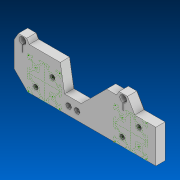
# Autodesk Inventor part: y-rear-V2
Saved by Autodesk Inventor 2021 (Build 250183000, 183)
## iProperties
Created: 2021-03-09
Part Number: y-rear-V2
Material: Generic
Document SubType Name: Modeling
Designer: Alex
Density: 1 g/cm^3
Appearance: Default
Author: Alex
## iProperties of the stored document _3DPrint.ipt
Created: 2021-03-16
Part Number: _3DPrint
Material: Generic
Document SubType Name: Modeling
Designer: Alex
Density: 1 g/cm^3
Appearance: Default
Author: Alex
Autodesk Inventor part; units mm, degrees
ref_plane "YZ Plane" through (0, 0, 0) normal (1, 0, 0) x (0, 1, 0)
ref_plane "XZ Plane" through (0, 0, 0) normal (0, 1, 0) x (-1, 0, 0)
ref_plane "XY Plane" through (0, 0, 0) normal (0, 0, 1) x (1, 0, 0)
sketch "v_slot_locations" plane through (0, 0, 0) normal (0, 0, 1) x (1, 0, 0)
  circle A0 centre (10, 10) radius 2.3 construction
  line L0 (13.9, 12.8393) -> (13.9, 7.1607) construction
  line L1 (12.8393, 13.9) -> (13.9, 12.8393) construction
  line L2 (7.1607, 13.9) -> (12.8393, 13.9) construction
  line L3 (3.7607, 17.3) -> (7.1607, 13.9) construction
  line L4 (1.8, 17.3) -> (3.7607, 17.3) construction
  line L5 (1.8, 22.7) -> (1.8, 17.3) construction
  line L6 (17.3, 1.8) -> (22.7, 1.8) construction
  line L7 (17.3, 3.7607) -> (17.3, 1.8) construction
  line L8 (13.9, 7.1607) -> (17.3, 3.7607) construction
  line L9 (0, 14.58) -> (0, 25.42) construction
  line L10 (1.185, 13.395) -> (0, 14.58) construction
  line L11 (1.8, 13.395) -> (1.185, 13.395) construction
  line L12 (1.8, 15.5) -> (1.8, 13.395) construction
  line L13 (3.4393, 15.5) -> (1.8, 15.5) construction
  line L14 (6.1, 12.8393) -> (3.4393, 15.5) construction
  line L15 (6.1, 10.21) -> (6.1, 12.8393) construction
  line L16 (6.31, 10) -> (6.1, 10.21) construction
  line L17 (6.1, 9.79) -> (6.31, 10) construction
  line L18 (6.1, 7.1607) -> (6.1, 9.79) construction
  line L19 (3.4393, 4.5) -> (6.1, 7.1607) construction
  line L20 (1.8, 4.5) -> (3.4393, 4.5) construction
  line L21 (1.8, 6.605) -> (1.8, 4.5) construction
  line L22 (1.185, 6.605) -> (1.8, 6.605) construction
  line L23 (0, 5.42) -> (1.185, 6.605) construction
  line L24 (0, 1.5) -> (0, 5.42) construction
  arc A1 (0, 1.5) -> (1.5, 0) centre (1.5, 1.5) ccw construction
  line L25 (5.42, 0) -> (1.5, 0) construction
  line L26 (6.605, 1.185) -> (5.42, 0) construction
  line L27 (6.605, 1.8) -> (6.605, 1.185) construction
  line L28 (4.5, 1.8) -> (6.605, 1.8) construction
  line L29 (4.5, 3.4393) -> (4.5, 1.8) construction
  line L30 (7.1607, 6.1) -> (4.5, 3.4393) construction
  line L31 (9.79, 6.1) -> (7.1607, 6.1) construction
  line L32 (10, 6.31) -> (9.79, 6.1) construction
  line L33 (10.21, 6.1) -> (10, 6.31) construction
  line L34 (12.8393, 6.1) -> (10.21, 6.1) construction
  line L35 (15.5, 3.4393) -> (12.8393, 6.1) construction
  line L36 (15.5, 1.8) -> (15.5, 3.4393) construction
  line L37 (13.395, 1.8) -> (15.5, 1.8) construction
  line L38 (13.395, 1.185) -> (13.395, 1.8) construction
  line L39 (14.58, 0) -> (13.395, 1.185) construction
  line L40 (25.42, 0) -> (14.58, 0) construction
  line L41 (0, 1.5) -> (0, 0) construction
  line L42 (0, 0) -> (1.5, 0) construction
  line L43 (0, 20) -> (40, 20) construction
  line L44 (20, 0) -> (20, 40) construction
  line L45 (33.9, 10.21) -> (33.9, 12.8393) construction
  line L46 (32.8393, 13.9) -> (27.1607, 13.9) construction
  line L47 (33.69, 10) -> (33.9, 10.21) construction
  line L48 (33.9, 9.79) -> (33.69, 10) construction
  line L49 (27.1607, 13.9) -> (26.1, 12.8393) construction
  line L50 (33.9, 7.1607) -> (33.9, 9.79) construction
  circle A2 centre (30, 10) radius 2.3 construction
  line L51 (30.21, 6.1) -> (32.8393, 6.1) construction
  line L52 (26.1, 12.8393) -> (26.1, 7.1607) construction
  line L53 (30, 6.31) -> (30.21, 6.1) construction
  line L54 (29.79, 6.1) -> (30, 6.31) construction
  line L55 (27.1607, 6.1) -> (29.79, 6.1) construction
  line L56 (33.9, 12.8393) -> (36.5607, 15.5) construction
  line L57 (38.2, 13.395) -> (38.815, 13.395) construction
  line L58 (36.2393, 17.3) -> (32.8393, 13.9) construction
  line L59 (38.2, 15.5) -> (38.2, 13.395) construction
  line L60 (38.815, 13.395) -> (40, 14.58) construction
  line L61 (38.2, 17.3) -> (36.2393, 17.3) construction
  line L62 (38.2, 22.7) -> (38.2, 17.3) construction
  line L63 (40, 14.58) -> (40, 25.42) construction
  line L64 (36.5607, 15.5) -> (38.2, 15.5) construction
  line L65 (38.815, 6.605) -> (38.2, 6.605) construction
  line L66 (40, 5.42) -> (38.815, 6.605) construction
  line L67 (36.5607, 4.5) -> (33.9, 7.1607) construction
  line L68 (38.2, 6.605) -> (38.2, 4.5) construction
  line L69 (38.2, 4.5) -> (36.5607, 4.5) construction
  line L70 (32.8393, 6.1) -> (35.5, 3.4393) construction
  line L71 (40, 1.5) -> (40, 5.42) construction
  line L72 (35.5, 3.4393) -> (35.5, 1.8) construction
  line L73 (35.5, 1.8) -> (33.395, 1.8) construction
  line L74 (33.395, 1.8) -> (33.395, 1.185) construction
  line L75 (33.395, 1.185) -> (34.58, 0) construction
  line L76 (34.58, 0) -> (38.5, 0) construction
  arc A3 (38.5, 0) -> (40, 1.5) centre (38.5, 1.5) ccw construction
  line L77 (22.7, 3.7607) -> (22.7, 1.8) construction
  line L78 (26.1, 7.1607) -> (22.7, 3.7607) construction
  line L79 (25.42, 0) -> (26.605, 1.185) construction
  line L80 (24.5, 3.4393) -> (27.1607, 6.1) construction
  line L81 (24.5, 1.8) -> (24.5, 3.4393) construction
  line L82 (26.605, 1.8) -> (24.5, 1.8) construction
  line L83 (26.605, 1.185) -> (26.605, 1.8) construction
  line L84 (6.1, 29.79) -> (6.1, 27.1607) construction
  line L85 (7.1607, 26.1) -> (12.8393, 26.1) construction
  line L86 (6.31, 30) -> (6.1, 29.79) construction
  line L87 (6.1, 30.21) -> (6.31, 30) construction
  line L88 (12.8393, 26.1) -> (13.9, 27.1607) construction
  line L89 (6.1, 32.8393) -> (6.1, 30.21) construction
  circle A4 centre (10, 30) radius 2.3 construction
  line L90 (9.79, 33.9) -> (7.1607, 33.9) construction
  line L91 (13.9, 27.1607) -> (13.9, 32.8393) construction
  line L92 (10, 33.69) -> (9.79, 33.9) construction
  line L93 (10.21, 33.9) -> (10, 33.69) construction
  line L94 (12.8393, 33.9) -> (10.21, 33.9) construction
  line L95 (6.1, 27.1607) -> (3.4393, 24.5) construction
  line L96 (1.8, 26.605) -> (1.185, 26.605) construction
  line L97 (3.7607, 22.7) -> (7.1607, 26.1) construction
  line L98 (1.8, 24.5) -> (1.8, 26.605) construction
  line L99 (1.185, 26.605) -> (0, 25.42) construction
  line L100 (1.8, 22.7) -> (3.7607, 22.7) construction
  line L101 (3.4393, 24.5) -> (1.8, 24.5) construction
  line L102 (1.185, 33.395) -> (1.8, 33.395) construction
  line L103 (0, 34.58) -> (1.185, 33.395) construction
  line L104 (3.4393, 35.5) -> (6.1, 32.8393) construction
  line L105 (1.8, 33.395) -> (1.8, 35.5) construction
  line L106 (1.8, 35.5) -> (3.4393, 35.5) construction
  line L107 (7.1607, 33.9) -> (4.5, 36.5607) construction
  line L108 (0, 38.5) -> (0, 34.58) construction
  line L109 (4.5, 36.5607) -> (4.5, 38.2) construction
  line L110 (4.5, 38.2) -> (6.605, 38.2) construction
  line L111 (6.605, 38.2) -> (6.605, 38.815) construction
  line L112 (6.605, 38.815) -> (5.42, 40) construction
  line L113 (5.42, 40) -> (1.5, 40) construction
  arc A5 (1.5, 40) -> (0, 38.5) centre (1.5, 38.5) ccw construction
  line L114 (17.3, 38.2) -> (22.7, 38.2) construction
  line L115 (17.3, 36.2393) -> (17.3, 38.2) construction
  line L116 (13.9, 32.8393) -> (17.3, 36.2393) construction
  line L117 (14.58, 40) -> (13.395, 38.815) construction
  line L118 (15.5, 36.5607) -> (12.8393, 33.9) construction
  line L119 (15.5, 38.2) -> (15.5, 36.5607) construction
  line L120 (13.395, 38.2) -> (15.5, 38.2) construction
  line L121 (25.42, 40) -> (14.58, 40) construction
  line L122 (13.395, 38.815) -> (13.395, 38.2) construction
  line L123 (38.815, 26.605) -> (40, 25.42) construction
  line L124 (38.2, 26.605) -> (38.815, 26.605) construction
  line L125 (38.2, 24.5) -> (38.2, 26.605) construction
  line L126 (36.5607, 24.5) -> (38.2, 24.5) construction
  line L127 (38.2, 22.7) -> (36.2393, 22.7) construction
  line L128 (36.2393, 22.7) -> (32.8393, 26.1) construction
  line L129 (33.9, 27.1607) -> (36.5607, 24.5) construction
  line L130 (33.9, 29.79) -> (33.9, 27.1607) construction
  line L131 (32.8393, 26.1) -> (27.1607, 26.1) construction
  circle A6 centre (30, 30) radius 2.3 construction
  line L132 (33.9, 30.21) -> (33.69, 30) construction
  line L133 (33.69, 30) -> (33.9, 29.79) construction
  line L134 (33.9, 32.8393) -> (33.9, 30.21) construction
  line L135 (38.815, 33.395) -> (38.2, 33.395) construction
  line L136 (40, 34.58) -> (38.815, 33.395) construction
  line L137 (40, 38.5) -> (40, 34.58) construction
  line L138 (38.2, 33.395) -> (38.2, 35.5) construction
  line L139 (38.2, 35.5) -> (36.5607, 35.5) construction
  arc A7 (40, 38.5) -> (38.5, 40) centre (38.5, 38.5) ccw construction
  line L140 (34.58, 40) -> (38.5, 40) construction
  line L141 (33.395, 38.815) -> (34.58, 40) construction
  line L142 (33.395, 38.2) -> (33.395, 38.815) construction
  line L143 (35.5, 38.2) -> (33.395, 38.2) construction
  line L144 (35.5, 36.5607) -> (35.5, 38.2) construction
  line L145 (32.8393, 33.9) -> (35.5, 36.5607) construction
  line L146 (36.5607, 35.5) -> (33.9, 32.8393) construction
  line L147 (30.21, 33.9) -> (32.8393, 33.9) construction
  line L148 (29.79, 33.9) -> (30, 33.69) construction
  line L149 (30, 33.69) -> (30.21, 33.9) construction
  line L150 (27.1607, 33.9) -> (29.79, 33.9) construction
  line L151 (24.5, 36.5607) -> (27.1607, 33.9) construction
  line L152 (26.605, 38.815) -> (26.605, 38.2) construction
  line L153 (25.42, 40) -> (26.605, 38.815) construction
  line L154 (26.605, 38.2) -> (24.5, 38.2) construction
  line L155 (24.5, 38.2) -> (24.5, 36.5607) construction
  line L156 (22.7, 36.2393) -> (22.7, 38.2) construction
  line L157 (26.1, 32.8393) -> (22.7, 36.2393) construction
  line L158 (26.1, 27.1607) -> (26.1, 32.8393) construction
  line L159 (27.1607, 26.1) -> (26.1, 27.1607) construction
  line L160 (-96.9, 10.21) -> (-96.9, 12.8393) construction
  line L161 (-95.8393, 13.9) -> (-90.1607, 13.9) construction
  line L162 (-96.69, 10) -> (-96.9, 10.21) construction
  line L163 (-96.9, 9.79) -> (-96.69, 10) construction
  line L164 (-90.1607, 13.9) -> (-89.1, 12.8393) construction
  line L165 (-96.9, 7.1607) -> (-96.9, 9.79) construction
  circle A8 centre (-93, 10) radius 2.3 construction
  line L166 (-93.21, 6.1) -> (-95.8393, 6.1) construction
  line L167 (-89.1, 12.8393) -> (-89.1, 7.1607) construction
  line L168 (-93, 6.31) -> (-93.21, 6.1) construction
  line L169 (-92.79, 6.1) -> (-93, 6.31) construction
  line L170 (-90.1607, 6.1) -> (-92.79, 6.1) construction
  line L171 (-96.9, 12.8393) -> (-99.5607, 15.5) construction
  line L172 (-101.2, 13.395) -> (-101.815, 13.395) construction
  line L173 (-99.2393, 17.3) -> (-95.8393, 13.9) construction
  line L174 (-101.2, 15.5) -> (-101.2, 13.395) construction
  line L175 (-101.815, 13.395) -> (-103, 14.58) construction
  line L176 (-101.2, 17.3) -> (-99.2393, 17.3) construction
  line L177 (-101.2, 22.7) -> (-101.2, 17.3) construction
  line L178 (-103, 14.58) -> (-103, 25.42) construction
  line L179 (-99.5607, 15.5) -> (-101.2, 15.5) construction
  line L180 (-101.815, 6.605) -> (-101.2, 6.605) construction
  line L181 (-103, 5.42) -> (-101.815, 6.605) construction
  line L182 (-99.5607, 4.5) -> (-96.9, 7.1607) construction
  line L183 (-101.2, 6.605) -> (-101.2, 4.5) construction
  line L184 (-101.2, 4.5) -> (-99.5607, 4.5) construction
  line L185 (-95.8393, 6.1) -> (-98.5, 3.4393) construction
  line L186 (-103, 1.5) -> (-103, 5.42) construction
  line L187 (-98.5, 3.4393) -> (-98.5, 1.8) construction
  line L188 (-98.5, 1.8) -> (-96.395, 1.8) construction
  line L189 (-96.395, 1.8) -> (-96.395, 1.185) construction
  line L190 (-96.395, 1.185) -> (-97.58, 0) construction
  line L191 (-97.58, 0) -> (-101.5, 0) construction
  arc A9 (-103, 1.5) -> (-101.5, 0) centre (-101.5, 1.5) ccw construction
  line L192 (-85.7, 1.8) -> (-80.3, 1.8) construction
  line L193 (-85.7, 3.7607) -> (-85.7, 1.8) construction
  line L194 (-89.1, 7.1607) -> (-85.7, 3.7607) construction
  line L195 (-88.42, 0) -> (-89.605, 1.185) construction
  line L196 (-87.5, 3.4393) -> (-90.1607, 6.1) construction
  line L197 (-87.5, 1.8) -> (-87.5, 3.4393) construction
  line L198 (-89.605, 1.8) -> (-87.5, 1.8) construction
  line L199 (-77.58, 0) -> (-88.42, 0) construction
  line L200 (-89.605, 1.185) -> (-89.605, 1.8) construction
  line L201 (-103, 1.5) -> (-103, 0) construction
  line L202 (-103, 0) -> (-101.5, 0) construction
  line L203 (-103, 20) -> (-63, 20) construction
  line L204 (-83, 0) -> (-83, 40) construction
  line L205 (-64.185, 13.395) -> (-63, 14.58) construction
  line L206 (-64.8, 13.395) -> (-64.185, 13.395) construction
  line L207 (-64.8, 15.5) -> (-64.8, 13.395) construction
  line L208 (-66.4393, 15.5) -> (-64.8, 15.5) construction
  line L209 (-64.8, 17.3) -> (-66.7607, 17.3) construction
  line L210 (-66.7607, 17.3) -> (-70.1607, 13.9) construction
  line L211 (-69.1, 12.8393) -> (-66.4393, 15.5) construction
  line L212 (-69.1, 10.21) -> (-69.1, 12.8393) construction
  line L213 (-70.1607, 13.9) -> (-75.8393, 13.9) construction
  circle A10 centre (-73, 10) radius 2.3 construction
  line L214 (-69.1, 9.79) -> (-69.31, 10) construction
  line L215 (-69.31, 10) -> (-69.1, 10.21) construction
  line L216 (-69.1, 7.1607) -> (-69.1, 9.79) construction
  line L217 (-64.185, 6.605) -> (-64.8, 6.605) construction
  line L218 (-63, 5.42) -> (-64.185, 6.605) construction
  line L219 (-63, 1.5) -> (-63, 5.42) construction
  line L220 (-64.8, 6.605) -> (-64.8, 4.5) construction
  line L221 (-64.8, 4.5) -> (-66.4393, 4.5) construction
  arc A11 (-64.5, 0) -> (-63, 1.5) centre (-64.5, 1.5) ccw construction
  line L222 (-68.42, 0) -> (-64.5, 0) construction
  line L223 (-69.605, 1.185) -> (-68.42, 0) construction
  line L224 (-69.605, 1.8) -> (-69.605, 1.185) construction
  line L225 (-67.5, 1.8) -> (-69.605, 1.8) construction
  line L226 (-67.5, 3.4393) -> (-67.5, 1.8) construction
  line L227 (-70.1607, 6.1) -> (-67.5, 3.4393) construction
  line L228 (-66.4393, 4.5) -> (-69.1, 7.1607) construction
  line L229 (-72.79, 6.1) -> (-70.1607, 6.1) construction
  line L230 (-73.21, 6.1) -> (-73, 6.31) construction
  line L231 (-73, 6.31) -> (-72.79, 6.1) construction
  line L232 (-75.8393, 6.1) -> (-73.21, 6.1) construction
  line L233 (-78.5, 3.4393) -> (-75.8393, 6.1) construction
  line L234 (-76.395, 1.185) -> (-76.395, 1.8) construction
  line L235 (-77.58, 0) -> (-76.395, 1.185) construction
  line L236 (-76.395, 1.8) -> (-78.5, 1.8) construction
  line L237 (-78.5, 1.8) -> (-78.5, 3.4393) construction
  line L238 (-80.3, 3.7607) -> (-80.3, 1.8) construction
  line L239 (-76.9, 7.1607) -> (-80.3, 3.7607) construction
  line L240 (-76.9, 12.8393) -> (-76.9, 7.1607) construction
  line L241 (-75.8393, 13.9) -> (-76.9, 12.8393) construction
  line L242 (-63, 14.58) -> (-63, 25.42) construction
  line L243 (-64.8, 22.7) -> (-64.8, 17.3) construction
  line L244 (-80.3, 36.2393) -> (-80.3, 38.2) construction
  line L245 (-78.5, 38.2) -> (-78.5, 36.5607) construction
  line L246 (-77.58, 40) -> (-76.395, 38.815) construction
  line L247 (-76.395, 38.815) -> (-76.395, 38.2) construction
  line L248 (-76.395, 38.2) -> (-78.5, 38.2) construction
  line L249 (-76.9, 32.8393) -> (-80.3, 36.2393) construction
  line L250 (-78.5, 36.5607) -> (-75.8393, 33.9) construction
  line L251 (-70.1607, 26.1) -> (-75.8393, 26.1) construction
  circle A12 centre (-73, 30) radius 2.3 construction
  line L252 (-72.79, 33.9) -> (-70.1607, 33.9) construction
  line L253 (-73, 33.69) -> (-72.79, 33.9) construction
  line L254 (-73.21, 33.9) -> (-73, 33.69) construction
  line L255 (-75.8393, 33.9) -> (-73.21, 33.9) construction
  line L256 (-76.9, 27.1607) -> (-76.9, 32.8393) construction
  line L257 (-75.8393, 26.1) -> (-76.9, 27.1607) construction
  line L258 (-63, 38.5) -> (-63, 34.58) construction
  line L259 (-67.5, 36.5607) -> (-67.5, 38.2) construction
  line L260 (-67.5, 38.2) -> (-69.605, 38.2) construction
  line L261 (-69.605, 38.2) -> (-69.605, 38.815) construction
  arc A13 (-63, 38.5) -> (-64.5, 40) centre (-64.5, 38.5) ccw construction
  line L262 (-68.42, 40) -> (-64.5, 40) construction
  line L263 (-69.605, 38.815) -> (-68.42, 40) construction
  line L264 (-69.1, 32.8393) -> (-69.1, 30.21) construction
  line L265 (-64.185, 33.395) -> (-64.8, 33.395) construction
  line L266 (-63, 34.58) -> (-64.185, 33.395) construction
  line L267 (-66.4393, 35.5) -> (-69.1, 32.8393) construction
  line L268 (-64.8, 35.5) -> (-66.4393, 35.5) construction
  line L269 (-64.8, 33.395) -> (-64.8, 35.5) construction
  line L270 (-70.1607, 33.9) -> (-67.5, 36.5607) construction
  line L271 (-64.8, 22.7) -> (-66.7607, 22.7) construction
  line L272 (-66.7607, 22.7) -> (-70.1607, 26.1) construction
  line L273 (-69.31, 30) -> (-69.1, 29.79) construction
  line L274 (-69.1, 30.21) -> (-69.31, 30) construction
  line L275 (-69.1, 29.79) -> (-69.1, 27.1607) construction
  line L276 (-69.1, 27.1607) -> (-66.4393, 24.5) construction
  line L277 (-66.4393, 24.5) -> (-64.8, 24.5) construction
  line L278 (-64.8, 24.5) -> (-64.8, 26.605) construction
  line L279 (-64.185, 26.605) -> (-63, 25.42) construction
  line L280 (-64.8, 26.605) -> (-64.185, 26.605) construction
  line L281 (-95.8393, 26.1) -> (-90.1607, 26.1) construction
  line L282 (-90.1607, 26.1) -> (-89.1, 27.1607) construction
  line L283 (-96.9, 29.79) -> (-96.9, 27.1607) construction
  line L284 (-96.69, 30) -> (-96.9, 29.79) construction
  circle A14 centre (-93, 30) radius 2.3 construction
  line L285 (-89.1, 27.1607) -> (-89.1, 32.8393) construction
  line L286 (-92.79, 33.9) -> (-93, 33.69) construction
  line L287 (-90.1607, 33.9) -> (-92.79, 33.9) construction
  line L288 (-96.9, 30.21) -> (-96.69, 30) construction
  line L289 (-93, 33.69) -> (-93.21, 33.9) construction
  line L290 (-96.9, 32.8393) -> (-96.9, 30.21) construction
  line L291 (-96.9, 27.1607) -> (-99.5607, 24.5) construction
  line L292 (-99.2393, 22.7) -> (-95.8393, 26.1) construction
  line L293 (-87.5, 36.5607) -> (-90.1607, 33.9) construction
  line L294 (-89.1, 32.8393) -> (-85.7, 36.2393) construction
  line L295 (-98.5, 38.2) -> (-96.395, 38.2) construction
  line L296 (-96.395, 38.2) -> (-96.395, 38.815) construction
  line L297 (-96.395, 38.815) -> (-97.58, 40) construction
  line L298 (-101.2, 35.5) -> (-99.5607, 35.5) construction
  line L299 (-98.5, 36.5607) -> (-98.5, 38.2) construction
  line L300 (-97.58, 40) -> (-101.5, 40) construction
  line L301 (-101.2, 33.395) -> (-101.2, 35.5) construction
  line L302 (-103, 34.58) -> (-101.815, 33.395) construction
  line L303 (-101.815, 33.395) -> (-101.2, 33.395) construction
  line L304 (-95.8393, 33.9) -> (-98.5, 36.5607) construction
  line L305 (-99.5607, 35.5) -> (-96.9, 32.8393) construction
  line L306 (-93.21, 33.9) -> (-95.8393, 33.9) construction
  line L307 (-103, 38.5) -> (-103, 34.58) construction
  arc A15 (-101.5, 40) -> (-103, 38.5) centre (-101.5, 38.5) ccw construction
  line L308 (-89.605, 38.815) -> (-89.605, 38.2) construction
  line L309 (-88.42, 40) -> (-89.605, 38.815) construction
  line L310 (-89.605, 38.2) -> (-87.5, 38.2) construction
  line L311 (-87.5, 38.2) -> (-87.5, 36.5607) construction
  line L312 (-77.58, 40) -> (-88.42, 40) construction
  line L313 (-85.7, 36.2393) -> (-85.7, 38.2) construction
  line L314 (-85.7, 38.2) -> (-80.3, 38.2) construction
  line L315 (-101.2, 26.605) -> (-101.815, 26.605) construction
  line L316 (-101.815, 26.605) -> (-103, 25.42) construction
  line L317 (-101.2, 24.5) -> (-101.2, 26.605) construction
  line L318 (-99.5607, 24.5) -> (-101.2, 24.5) construction
  line L319 (-101.2, 22.7) -> (-99.2393, 22.7) construction
  point P0 (0, 0)
  dimension "d3" = 1.5
  dimension "d4" = 4.6
  dimension "d5" = 1.5
  dimension "d7" = 45
  dimension "d8" = 2.105
  dimension "d9" = 1.6393
  dimension "d10" = 1.185
  dimension "d11" = 45
  dimension "d12" = 0.615
  dimension "d13" = 45
  dimension "d16" = 135
  dimension "d17" = 135
  dimension "d18" = 45
  dimension "d19" = 1.5
  dimension "d20" = 2.6293
  dimension "d21" = 2.6293
  dimension "d23" = 45
  dimension "d24" = 2.105
  dimension "d25" = 10.84
  dimension "d26" = 135
  dimension "d27" = 135
  dimension "d28" = 2.6607
  dimension "d29" = 45
  dimension "d30" = 1.185
  dimension "d33" = 0.21
  dimension "d34" = 1.5
  dimension "d35" = 3.9
  dimension "d36" = 3.9
  dimension "d37" = 135
  dimension "d38" = 1.0607
  dimension "d39" = 1.185
  dimension "d40" = 0.615
  dimension "d41" = 1.6393
  dimension "d42" = 1.8
  dimension "d43" = 0.21
  dimension "d44" = 135
  dimension "d45" = 5.4
  dimension "d46" = 1.9607
  dimension "d47" = 1.8
  dimension "d49" = 5.4
  dimension "d50" = 1.8
  dimension "d51" = 40
  dimension "d52" = 40
  dimension "d98" = 13.395
  dimension "d99" = 10
  dimension "d100" = 10
  dimension "d101" = 6.605
  dimension "d102" = 10
  dimension "d103" = 13.395
  dimension "d104" = 1.5
  dimension "d105" = 4.6
  dimension "d106" = 1.5
  dimension "d107" = 45
  dimension "d108" = 2.105
  dimension "d109" = 1.6393
  dimension "d110" = 1.185
  dimension "d111" = 45
  dimension "d112" = 0.615
  dimension "d113" = 45
  dimension "d114" = 135
  dimension "d115" = 135
  dimension "d116" = 45
  dimension "d117" = 1.5
  dimension "d118" = 2.6293
  constraints: 640 end point, 244 symmetric about line, 30 vertical, 28 horizontal, 18 equal length, 16 centre point, 16 point on circle, 7 collinear, 4 midpoint, 4 tangent, 2 perpendicular, 1 coincident, 12 other
  measures "d3" radius of A1
  measures "d4" diameter of A0
  measures "d5" distance between parallel lines of L30 L19
  measures "d7" angle of L25 L26
  measures "d8" distance of L29.end L28.end
  measures "d9" distance of L30.end L29.end
  measures "d10" horizontal distance of L27.end L26.end
  measures "d11" angle of L24 L23
  measures "d12" distance of L28.end L27.end
  measures "d13" angle of L30 L29
  measures "d16" angle of L18 L17
  measures "d17" angle of L15 L16
  measures "d18" angle of L0 L1
  measures "d19" distance between parallel lines of L3 L14
  measures "d20" distance of L18.start L17.start
  measures "d21" distance of L15.start L15.end
  measures "d23" angle of L11 L10
  measures "d24" distance of L12.start L11.start
  measures "d25" distance of L10.end L9.end
  measures "d26" angle of L31 L32
  measures "d27" angle of L34 L33
  measures "d28" horizontal distance of L31.end L30.end
  measures "d29" angle of L40 L39
  measures "d30" horizontal distance of L39.start L39.end
  measures "d33" horizontal distance of L32.start L31.start
  measures "d34" distance between parallel lines of L8 L35
  measures "d35" distance from line of L0 A0.centre
  measures "d36" distance from line of L2 A0.centre
  measures "d37" angle of L35 L36
  measures "d38" horizontal distance of L2.end L1.end
  measures "d39" horizontal distance of L11.end L10.end
  measures "d40" distance of L11.start L11.end
  measures "d41" distance of L14.end L12.start
  measures "d42" distance between parallel lines of L13 L4
  measures "d43" horizontal distance of L16.start L15.start
  measures "d44" angle of L2 L3
  measures "d45" distance of L6.start L6.end
  measures "d46" distance of L7.start L6.start
  measures "d47" distance between parallel lines of L7 L36
  measures "d49" distance of L5.start L4.start
  measures "d50" distance between parallel lines of L9 L5
  measures "d51" distance of L43.start L43.end
  measures "d52" distance of L44.start L44.end
  measures "d98" distance between parallel lines of L38 L24
  measures "d99" distance from line of A0.centre L24
  measures "d100" distance from line of L32.start L24
  measures "d101" distance between parallel lines of L27 L24
  measures "d102" distance from line of A0.centre L25
  measures "d103" distance between parallel lines of L11 L25
  measures "d104" radius of A9
  measures "d105" diameter of A8
  measures "d106" distance between parallel lines of L185 L182
  measures "d107" angle of L191 L190
  measures "d108" distance of L187.end L188.end
  measures "d109" distance of L185.end L187.end
  measures "d110" horizontal distance of L189.end L190.end
  measures "d111" angle of L186 L181
  measures "d112" distance of L188.end L189.end
  measures "d113" angle of L185 L187
  measures "d114" angle of L165 L163
  measures "d115" angle of L160 L162
  measures "d116" angle of L167 L164
  measures "d117" distance between parallel lines of L173 L171
  measures "d118" distance of L165.start L165.end
sketch "Sketch2" plane through (0, 0, 0) normal (0, 0, 1) x (1, 0, 0)
  line L0 (-103, 0) -> (50, 0)
  line L1 (50, 0) -> (50, 40)
  line L2 (50, 40) -> (24.8564, 40)
  line L3 (24.8564, 40) -> (16.1962, 55)
  line L4 (16.1962, 55) -> (6.1962, 55)
  line L5 (6.1962, 55) -> (3.3094, 50)
  line L6 (3.3094, 50) -> (-100.9171, 50)
  line L7 (-100.9171, 50) -> (-103.8038, 55)
  line L8 (-103.8038, 55) -> (-113.8038, 55)
  line L9 (-113.8038, 55) -> (-119, 46)
  line L10 (-119, 46) -> (-119, 16)
  line L11 (-119, 16) -> (-103, 0)
  line L12 (-152.8, 0) -> (83.8, 0) projected
  circle A0 centre (-73, 30) radius 2.3 construction
  circle A1 centre (-93, 10) radius 2.3 construction
  circle A2 centre (10, 10) radius 2.3 construction
  circle A3 centre (30, 30) radius 2.3 construction
  arc A4 (-108.4288, 45.9423) -> (-109.1788, 45.9423) centre (-108.8038, 50) ccw
  arc A5 (11.5712, 45.9423) -> (10.8212, 45.9423) centre (11.1962, 50) ccw
  line L13 (-108.8038, 55) -> (-108.8038, 50) construction
  line L14 (11.1962, 55) -> (11.1962, 50) construction
  line L15 (-109.1788, 45.9423) -> (-109.1788, 37.9423)
  line L16 (-109.1788, 37.9423) -> (-108.4288, 37.9423)
  line L17 (-108.4288, 37.9423) -> (-108.4288, 45.9423)
  line L18 (10.8212, 45.9423) -> (10.8212, 37.9423)
  line L19 (10.8212, 37.9423) -> (11.5712, 37.9423)
  line L20 (11.5712, 37.9423) -> (11.5712, 45.9423)
  line L21 (40, 14.58) -> (40, 25.42) construction
  line L22 (25.42, 40) -> (14.58, 40) construction
  line L23 (-103, 1.5) -> (-103, 0) construction
  line L24 (-48.8038, 50) -> (-48.8038, 0) construction
  line L25 (-63.9171, 50) -> (-58.8038, 20)
  line L26 (-58.8038, 20) -> (-38.8038, 20)
  line L27 (-38.8038, 20) -> (-8.8038, 50)
  circle A6 centre (-53.8038, 10) radius 1.7
  circle A7 centre (-43.8038, 10) radius 1.7
  line L28 (-53.8038, 10) -> (-43.8038, 10) construction
  circle A8 centre (-93, 10) radius 2.75
  circle A9 centre (-73, 30) radius 2.75
  circle A10 centre (10, 10) radius 2.75
  circle A11 centre (30, 30) radius 2.75
  point P0 (0, 0)
  dimension "d154" = 5
  dimension "d155" = 8.15
  dimension "d156" = 0.75
  dimension "d157" = 8
  dimension "d160" = 10
  dimension "d161" = 10
  dimension "d162" = 120
  dimension "d163" = 50
  dimension "d164" = 150
  dimension "d165" = 45
  dimension "d166" = 16
  dimension "d167" = 9
  dimension "d168" = 5
  dimension "d169" = 120
  dimension "d258" = 60
  dimension "d261" = 30
  dimension "d262" = 37
  dimension "d263" = 20
  dimension "d264" = 135
  dimension "d265" = 3.4
  dimension "d266" = 3.4
  dimension "d267" = 10
  dimension "d268" = 10
  dimension "d274" = 5.5
  constraints: 50 end point, 8 centre point, 7 perpendicular, 6 point on line, 5 vertical, 4 coincident, 4 equal length, 4 equal radius, 4 parallel, 4 point on circle, 3 horizontal, 3 midpoint, 2 collinear, 2 symmetric about line, 2 other
  measures "d154" distance of L13.start L13.end
  measures "d155" diameter of A4
  measures "d156" distance of L15.end L16.end
  measures "d157" distance of L16.end L17.end
  measures "d160" distance of L7.end L8.end
  measures "d161" distance between parallel lines of L21 L1
  measures "d162" angle of L2 L3
  measures "d163" distance between parallel lines of L12 L6
  measures "d164" angle of L10 L9
  measures "d165" angle of L12 L11
  measures "d166" horizontal distance of L10.end L0.start
  measures "d167" vertical distance of L8.end L9.end
  measures "d168" distance between parallel lines of L6 L8
  measures "d169" distance between parallel lines of L13 L14
  measures "d258" distance from line of L24 L14.end
  measures "d261" distance between parallel lines of L6 L26
  measures "d262" distance of L25.start L6.end
  measures "d263" distance of L25.end L26.end
  measures "d264" angle of L6 L27
  measures "d265" diameter of A6
  measures "d266" diameter of A7
  measures "d267" distance from line of L12 L28.start
  measures "d268" distance of L28.end L28.start
  measures "d274" diameter of A8
extrude "base" add sketch "Sketch2" against normal blind 12 contours L11 L10 L9 L8 L7 L6 L25 L26 L27 L5 L4 L3 L2 L1 L0
sketch "Sketch13" plane through (0, 0, -12) normal (0, 0, -1) x (-1, 0, 0)
  arc A0 (-10.8212, 45.9423) -> (-11.5712, 45.9423) centre (-11.1962, 50) ccw projected
  line L0 (-10.8212, 45.9423) -> (-10.8212, 37.9423) projected
  line L1 (-11.5712, 37.9423) -> (-11.5712, 45.9423) projected
  line L2 (-10.8212, 37.9423) -> (-11.5712, 37.9423) projected
  arc A1 (109.1788, 45.9423) -> (108.4288, 45.9423) centre (108.8038, 50) ccw projected
  line L3 (109.1788, 45.9423) -> (109.1788, 37.9423) projected
  line L4 (108.4288, 37.9423) -> (108.4288, 45.9423) projected
  line L5 (109.1788, 37.9423) -> (108.4288, 37.9423) projected
  point P0 (0, 0)
extrude "rod_fills" add sketch "Sketch13" against normal blind 2
sketch "Sketch14" plane through (0, 0, 0) normal (0, 0, 1) x (1, 0, 0)
  circle A0 centre (-53.8038, 10) radius 1.7 projected
  line L0 (-50.3397, 10) -> (-52.0718, 7)
  line L1 (-52.0718, 7) -> (-55.5359, 7)
  line L2 (-55.5359, 7) -> (-57.2679, 10)
  line L3 (-57.2679, 10) -> (-55.5359, 13)
  line L4 (-55.5359, 13) -> (-52.0718, 13)
  line L5 (-52.0718, 13) -> (-50.3397, 10)
  circle A1 centre (-43.8038, 10) radius 1.7 projected
  line L6 (-42.0718, 13) -> (-40.3397, 10)
  line L7 (-40.3397, 10) -> (-42.0718, 7)
  line L8 (-42.0718, 7) -> (-45.5359, 7)
  line L9 (-45.5359, 7) -> (-47.2679, 10)
  line L10 (-47.2679, 10) -> (-45.5359, 13)
  line L11 (-45.5359, 13) -> (-42.0718, 13)
  point P0 (0, 0)
  dimension "d270" = 6
  dimension "d271" = 6
  constraints: 24 end point, 2 coincident, 2 horizontal, 26 other
  measures "d270" distance between parallel lines of L1 L4
  measures "d271" distance between parallel lines of L8 L11
extrude "Extrusion10" cut sketch "Sketch14" against normal blind 3 contours A0 | L0 L1 L2 L3 L4 L5 | A1 | L6 L7 L8 L9 L10 L11
chamfer "Chamfer10" distance 1 angle 45 15 edges at (37.4282, 40, -12) (50, 20, -12) (20.5263, 47.5, -12) (11.1962, 55, -12) (4.7528, 52.5, -12) (-2.7472, 50, -12) (-23.8038, 35, -12) (-48.8038, 20, -12) (-61.3605, 35, -12) (-82.4171, 50, -12) (-102.3605, 52.5, -12) (-108.8038, 55, -12) (-116.4019, 50.5, -12) (-119, 31, -12) (-111, 8, -12)
body "Solid1"
